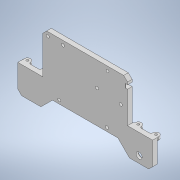
# Autodesk Inventor part: Driver Board Mount
Saved by Autodesk Inventor 2022 (Build 260153000, 153)
## iProperties
Created: 2022-05-29
Part Number: Driver Board Mount
Material: Generic
Document SubType Name: Modeling
Designer: Nick
Density: 1 g/cm^3
Appearance: Default
Author: Nick
Autodesk Inventor part; units mm, degrees
ref_plane "YZ Plane" through (0, 0, 0) normal (1, 0, 0) x (0, 1, 0)
ref_plane "XZ Plane" through (0, 0, 0) normal (0, 1, 0) x (-1, 0, 0)
sketch "Sketch1" plane through (0, 0, 0) normal (0, 0, 1) x (1, 0, 0)
  line L0 (-32.5, 0) -> (0, 0)
  line L1 (0, 0) -> (0, 54.05)
  line L2 (0, 54.05) -> (110, 54.05)
  line L3 (110, 54.05) -> (110, 0)
  line L4 (110, 0) -> (142.5, 0)
  line L5 (142.5, 0) -> (142.5, -35)
  line L6 (142.5, -35) -> (112.5, -35)
  line L7 (112.5, -35) -> (97.5, -20)
  line L8 (97.5, -20) -> (12.5, -20)
  line L9 (12.5, -20) -> (-2.5, -35)
  line L10 (-2.5, -35) -> (-32.5, -35)
  line L11 (-32.5, -35) -> (-32.5, 0)
  dimension "d0" = 135
  dimension "d1" = 135
  dimension "d2" = 110
  dimension "d3" = 54.05
  dimension "d4" = 35
  dimension "d5" = 32.5
  dimension "d6" = 20
  dimension "d7" = 30
  constraints: 24 end point, 4 collinear, 4 horizontal, 2 parallel, 2 perpendicular, 2 vertical, 1 coincident
  measures "d0" angle of L10 L9
  measures "d1" angle of L6 L7
  measures "d2" distance of L1.end L2.end
  measures "d3" distance of L0.end L1.end
  measures "d4" distance of L10.end L0.start
  measures "d5" distance of L0.start L0.end
  measures "d6" distance between parallel lines of L0 L8
  measures "d7" distance of L5.end L6.end
extrude "Extrusion1" add sketch "Sketch1" along normal blind 6
chamfer "Chamfer1" distance 5 angle 45 4 edges at (0, 54.05, 3) (110, 54.05, 3) (-32.5, -35, 3) (142.5, -35, 3)
sketch "Sketch2" plane through (110, 0, 0) normal (0, 1, 0) x (1, 0, 0)
  circle A0 centre (-138.5, 2.5) radius 1.5
  circle A1 centre (-115.5, 2.5) radius 1.5
  line L0 (-142.5, 0) -> (-142.5, -6) projected
  line L1 (-110, 0) -> (-142.5, 0) projected
  circle A2 centre (-138.5, 2.5) radius 4
  line L2 (-142.5, 0) -> (-112.5, 0) projected
  arc A3 (-142.5, 0) -> (-142.3846, 1.5461) centre (-144.8125, 0.95) ccw
  arc A4 (-134.5, 2.5) -> (-132, 0) centre (-132, 2.5) ccw
  arc A5 (-122, 0) -> (-119.5, 2.5) centre (-122, 2.5) ccw
  arc A6 (-111.5, 2.5) -> (-109, 0) centre (-109, 2.5) ccw
  circle A7 centre (-115.5, 2.5) radius 4
  line L3 (-109, 0) -> (-112.3775, 0)
  line L4 (-112.5, 0) -> (-97.5, 0) projected
  point P0 (-122, 0)
  point P1 (-132, 0)
  point P2 (-118.6225, 0)
  point P3 (-112.3775, 0)
  dimension "d13" = 3
  dimension "d14" = 3
  dimension "d15" = 4
  dimension "d16" = 27
  dimension "d17" = 2.5
  dimension "d18" = 8
  constraints: 13 point on circle, 8 centre point, 7 tangent, 4 equal radius, 4 point on line, 2 coincident, 2 end point, 2 horizontal alignment
  measures "d13" diameter of A1
  measures "d14" diameter of A0
  measures "d15" distance from line of L0 A0.centre
  measures "d16" distance from line of A1.centre L0
  measures "d17" distance from line of L1 A1.centre
  measures "d18" diameter of A2
extrude "Extrusion2" add sketch "Sketch2" against normal blind 4 contours L1 A2 A4 | L1 A7 A6 L3 | L1 A7 | L1 A5 A7 | L1 A2 | L1 A3 A2 picked at (-115.6011, 0.337) picked at (-138.4397, 0.337)
sketch "Sketch3" plane through (0, 0, 0) normal (0, 0, -1) x (-1, 0, 0)
  line L0 (-105, 54.05) -> (-5, 54.05) projected
  line L1 (0, 49.05) -> (0, 0) projected
  line L2 (-110, 0) -> (-110, 49.05) projected
  point P0 (-84, 48.55)
  point P1 (-26, 48.55)
  dimension "d21" = 5.5
  dimension "d22" = 26
  dimension "d23" = 26
  constraints: 1 horizontal alignment
  measures "d21" distance from line of L0 point (-26, 48.55)
  measures "d22" distance from line of L1 point (-26, 48.55)
  measures "d23" distance from line of L2 point (-84, 48.55)
hole "Hole1" at (84, 48.55, 0) at (26, 48.55, 0) direction (0, 0, 1) diameter 4 depth 24
sketch "Sketch4" plane through (12.5, -20, 0) normal (0, -1, 0) x (1, 0, 0)
  line L0 (74, 1.5) -> (72.5, 1.5)
  line L1 (72.5, 1.5) -> (72.5, 4.5)
  line L2 (72.5, 4.5) -> (74, 4.5)
  line L3 (74, 4.5) -> (74, 1.5)
  line L4 (77, 1.5) -> (77, 4.5)
  line L5 (-15, 0) -> (-15, 6) projected
  line L6 (85, 0) -> (85, 6) projected
  line L7 (53.5, 1.5) -> (52, 1.5)
  line L8 (52, 1.5) -> (52, 4.5)
  line L9 (52, 4.5) -> (53.5, 4.5)
  line L10 (53.5, 4.5) -> (53.5, 1.5)
  line L11 (56.5, 1.5) -> (56.5, 4.5)
  point P0 (-12.5, 0)
  point P1 (72.5, 3)
  point P2 (-15, 3)
  point P3 (77, 3)
  point P4 (74, 3)
  point P5 (53.5, 3)
  point P6 (56.5, 3)
  dimension "d31" = 1.5
  dimension "d32" = 3
  dimension "d33" = 3
  dimension "d35" = 8
  dimension "d36" = 1.5
  dimension "d37" = 3
  dimension "d38" = 3
  dimension "d39" = 16
  constraints: 20 end point, 6 horizontal alignment, 6 midpoint, 4 parallel, 2 horizontal, 2 perpendicular, 2 vertical
  measures "d31" distance of L1.end L2.end
  measures "d32" distance of L0.end L1.end
  measures "d33" distance between parallel lines of L4 L3
  measures "d35" distance between parallel lines of L6 L4
  measures "d36" distance of L7.start L7.end
  measures "d37" distance of L7.end L8.end
  measures "d38" distance between parallel lines of L10 L11
  measures "d39" distance between parallel lines of L1 L11
revolve "Revolution1" cut sketch "Sketch4" angle 360 about axis through (89.5, -20, 1.5) along (0, 0, 1) contours L0 L1 L2 L3
revolve "Revolution2" cut sketch "Sketch4" angle 360 about axis through (69, -20, 1.5) along (0, 0, 1) contours L7 L8 L9 L10
ref_plane "Work Plane1" through (55, 0, 6) normal (1, 0, 0) x (0, 0, -1)
mirror "Mirror1" about plane through (55, 0, 6) normal (1, 0, 0) of "Extrusion2"
sketch "Sketch5" plane through (0, 0, 6) normal (0, 0, 1) x (1, 0, 0)
  circle A0 centre (101.2237, 19.6209) radius 1.6
  circle A1 centre (70.2706, 22.6087) radius 1.6
  circle A2 centre (21.34, -15.4078) radius 1.6
  circle A3 centre (83.2562, -15.291) radius 1.6
  circle A4 centre (6.3179, 48.8175) radius 1.6
  circle A5 centre (70.2706, 22.6087) radius 4
  circle A6 centre (101.2237, 19.6209) radius 4
  circle A7 centre (83.2562, -15.291) radius 4
  circle A8 centre (21.34, -15.4078) radius 4
  circle A9 centre (6.3179, 48.8175) radius 4
  line L0 (109, 0) -> (109, -4) projected
  line L1 (12.5, -20) -> (97.5, -20) projected
  line L2 (110, 0) -> (97.5, -20)
  circle A10 centre (26, 48.55) radius 2
  circle A11 centre (84, 48.55) radius 2
  circle A12 centre (26, 48.55) radius 4
  circle A13 centre (84, 48.55) radius 4
  circle A14 centre (84, 48.55) radius 2
  circle A15 centre (26, 48.55) radius 2
  line L3 (105, 54.05) -> (110, 49.05) projected
  line L4 (105, 54.05) -> (5, 54.05) projected
  line L5 (0, 49.05) -> (5, 54.05) projected
  line L6 (0, 49.05) -> (0, 0) projected
  line L7 (0, 0) -> (-32.5, 0) projected
  line L8 (-32.5, 0) -> (-32.5, -30) projected
  line L9 (-27.5, -35) -> (-2.5, -35) projected
  line L10 (-2.5, -35) -> (12.5, -20) projected
  line L11 (12.5, -20) -> (97.5, -20) projected
  line L12 (97.5, -20) -> (112.5, -35) projected
  line L13 (112.5, -35) -> (137.5, -35) projected
  line L14 (142.5, -30) -> (142.5, 0) projected
  line L15 (142.5, 0) -> (110, 0) projected
  line L16 (110, 0) -> (110, 49.05) projected
  line L17 (0, 49.05) -> (5, 54.05) projected
  line L18 (105, 54.05) -> (5, 54.05) projected
  line L19 (105, 54.05) -> (110, 49.05) projected
  line L20 (142.5, -30) -> (137.5, -35) projected
  line L21 (-27.5, -35) -> (-32.5, -30) projected
  circle A16 centre (6.3179, 48.8175) radius 1.6
  circle A17 centre (21.34, -15.4078) radius 1.6
  circle A18 centre (70.2706, 22.6087) radius 1.6
  circle A19 centre (101.2237, 19.6209) radius 1.6
  circle A20 centre (83.2562, -15.291) radius 1.6
  line L22 (110, 0) -> (110, 49.05) projected
  line L23 (0, 49.05) -> (0, 0) projected
  dimension "d41" = 8
  dimension "d82" = 5.5
  dimension "d83" = 5.5
  dimension "d84" = 26
  dimension "d85" = 26
  constraints: 21 centre point, 5 coincident, 2 end point, 10 other
  measures "d41" diameter of A9
  measures "d82" distance from line of L18 A10.centre
  measures "d83" distance from line of L18 A11.centre
  measures "d84" distance from line of L22 A11.centre
  measures "d85" distance from line of L23 A10.centre
hole "Hole2" at (6.3179, 48.8175, 6) at (70.2706, 22.6087, 6) at (101.2237, 19.6209, 6) at (83.2562, -15.291, 6) at (21.34, -15.4078, 6) direction (0, 0, -1) diameter 4 depth 24
sketch "Sketch6" plane through (0, 0, 0) normal (0, 0, -1) x (-1, 0, 0)
  line L0 (-110, 0) -> (-110, 49.05) projected
  line L1 (-110, 46.05) -> (-107, 46.05)
  line L2 (-107, 46.05) -> (-90, 46.05)
  line L3 (-90, 46.05) -> (-90, 10)
  line L4 (-90, 10) -> (-95, 10)
  line L5 (-95, 10) -> (-95, 41.05)
  line L6 (-95, 41.05) -> (-110, 41.05)
  line L7 (-110, 0) -> (-110, 49.05) projected
  line L8 (-12.5, -20) -> (-97.5, -20) projected
  line L9 (-107, 46.05) -> (-107, 41.05)
  point P0 (0, 0)
  dimension "d49" = 30
  dimension "d50" = 5
  dimension "d51" = 5
  dimension "d55" = 15
  dimension "d68" = 3
  dimension "d69" = 3
  constraints: 14 end point, 7 perpendicular, 3 point on line, 1 parallel
  measures "d49" distance between parallel lines of L8 L4
  measures "d50" distance of L3.end L4.end
  measures "d51" distance between parallel lines of L2 L6
  measures "d55" distance of L5.end L6.end
  measures "d68" distance from line of L0.end L1
  measures "d69" distance between parallel lines of L0 L9
extrude "Extrusion3" cut sketch "Sketch6" against normal blind 3
extrude "Extrusion4" cut sketch "Sketch6" against normal through all contours L0 L1 L9 L6
fillet "Fillet1" radius 4 1 edges at (95, 41.05, 1.5)
fillet "Fillet2" radius 9 1 edges at (90, 46.05, 1.5)
chamfer "Chamfer2" distance 2 angle 45 2 edges at (92.5, 10, 0) (107, 43.55, 3)
sketch "Sketch7" plane through (0, 0, 0) normal (0, 0, -1) x (-1, 0, 0)
  circle A0 centre (-125, -26) radius 4
  circle A1 centre (-125, -26) radius 5 construction
  circle A2 centre (-125, -26) radius 9 construction
  line L0 (-112.5, -35) -> (-137.5, -35) projected
  circle A3 centre (-125, -26) radius 7.5
  point P0 (0, 0)
  point P1 (-125, -35)
  dimension "d70" = 8
  dimension "d71" = 10
  dimension "d72" = 18
  dimension "d75" = 15
  constraints: 4 centre point, 3 coincident, 1 midpoint, 1 tangent, 1 vertical alignment
  measures "d70" diameter of A0
  measures "d71" diameter of A1
  measures "d72" diameter of A2
  measures "d75" diameter of A3
extrude "Extrusion5" cut sketch "Sketch7" against normal through all contours A0
extrude "Extrusion6" cut sketch "Sketch7" against normal blind 3 contours A0 | A3
equation "\"d51\" = d50"
equation "\"d61\" = d60 + d50"
equation "\"MotorHeight\" = MotorHeightBase"
equation "\"d60\" = 4"
equation "\"MotorHeightBase\" = 28"
body "Solid1"
